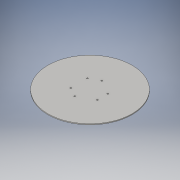
# Autodesk Inventor part: Base
Saved by Autodesk Inventor 2016 (Build 200138000, 138)
## iProperties
Created: 2015-10-01
Part Number: Base
Material: Generic
Document SubType Name: Modeling
Designer: Mack
Density: 1 g/cm^3
Appearance: Default
Author: Mack
Autodesk Inventor part; units mm, degrees
ref_plane "YZ Plane" through (0, 0, 0) normal (1, 0, 0) x (0, 1, 0)
ref_plane "XZ Plane" through (0, 0, 0) normal (0, 1, 0) x (-1, 0, 0)
ref_plane "XY Plane" through (0, 0, 0) normal (0, 0, 1) x (1, 0, 0)
sketch "Sketch1" plane through (0, 0, 0) normal (0, 1, 0) x (-1, 0, 0)
  circle A0 centre (0, 0) radius 152.4
  dimension "d0" = 304.8
  constraints: 1 centre point, 1 coincident
  measures "d0" diameter of A0
extrude "Extrusion1" add sketch "Sketch1" along normal blind 3.175
sketch "Sketch2" plane through (0, 3.175, 0) normal (0, 1, 0) x (1, 0, 0)
  point P0 (0, 0)
  point P1 (45.72, -19.05)
  point P2 (45.72, 19.05)
  point P3 (-39.3578, 30.0697)
  point P4 (-6.3622, 49.1197)
  point P5 (-6.3622, -49.1197)
  point P6 (-39.3578, -30.0697)
  dimension "d4" = 45.72
  dimension "d5" = 19.05
  dimension "d6" = 19.05
  dimension "d7" = 45.72
  dimension "d10" = 360
  constraints: 7 other
  measures "d4" horizontal distance of point (0, 0) point (45.72, -19.05)
  measures "d5" vertical distance of point (0, 0) point (45.72, -19.05)
  measures "d6" vertical distance of point (0, 0) point (45.72, 19.05)
  measures "d7" horizontal distance of point (0, 0) point (45.72, 19.05)
hole "Hole1" at (45.72, 3.175, 19.05) at (45.72, 3.175, -19.05) at (-39.3578, 3.175, -30.0697) at (-6.3622, 3.175, -49.1197) at (-6.3622, 3.175, 49.1197) at (-39.3578, 3.175, 30.0697) direction (0, -1, 0) diameter 5 end through all
body "Solid1"
